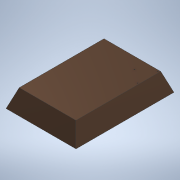
# Autodesk Inventor part: Base
Saved by Autodesk Inventor 2022 (Build 260153000, 153)
## iProperties
Created: 2021-06-28
Part Number: Base
Material: Generic
Document SubType Name: Modeling
Designer: Prajwal Patil
Density: 1 g/cm^3
Appearance: Default
Author: Prajwal Patil
Autodesk Inventor part; units mm, degrees
ref_plane "YZ Plane" through (0, 0, 0) normal (1, 0, 0) x (0, 1, 0)
ref_plane "XZ Plane" through (0, 0, 0) normal (0, 1, 0) x (-1, 0, 0)
ref_plane "XY Plane" through (0, 0, 0) normal (0, 0, 1) x (1, 0, 0)
sketch "Sketch1" plane through (0, 0, 0) normal (0, 1, 0) x (-1, 0, 0)
  line L0 (0, 0) -> (0, -129.54)
  line L1 (0, 0) -> (99.06, 0)
  line L2 (99.06, 0) -> (99.06, -129.54)
  line L3 (99.06, -129.54) -> (0, -129.54)
  line L4 (140.0707, 45.2128) -> (-215.5629, 45.2128)
  line L5 (-215.5629, 45.2128) -> (-215.5629, -504.8339)
  line L6 (-215.5629, -504.8339) -> (140.0707, -504.8339)
  line L7 (140.0707, -504.8339) -> (140.0707, 45.2128)
  dimension "d0" = 129.54
  dimension "d1" = 99.06
  constraints: 16 end point, 3 perpendicular, 2 horizontal, 2 parallel, 1 vertical
  measures "d0" distance of L0.start L0.end
  measures "d1" distance of L0.start L1.end
extrude "Extrusion1" add sketch "Sketch1" against normal blind 101.6 contours L1 L2 L3 L0 | L7 L6 L5 L4
draft "FaceDraft1" angle -20 pull direction (0, -1, 0) faces at (215.5629, -33.8667, -138.1361) (-21.5262, -33.8667, 45.2128) fixed edges at (215.5629, -101.6, -229.8106) (37.7461, -101.6, 45.2128)
draft "FaceDraft2" angle -20 pull direction (0, -1, 0) faces at (-140.0707, -67.7333, -150.4626) (84.6919, -67.7333, -504.8339) fixed edges at (-140.0707, 0, -248.3003) (37.7461, -101.6, -504.8339)
sketch "Sketch2" plane through (0, 0, 0) normal (0, 1, 0) x (1, 0, 0)
  line L0 (178.5835, 467.8546) -> (215.5629, 504.8339) projected
  line L1 (178.5835, 467.8546) -> (79.5235, 467.8546)
  line L2 (79.5235, 467.8546) -> (79.5235, 338.3146)
  line L3 (79.5235, 338.3146) -> (178.5835, 338.3146)
  line L4 (178.5835, 338.3146) -> (178.5835, 467.8546)
  line L5 (178.5835, 338.3146) -> (178.5835, 346.4426)
  line L6 (178.5835, -8.2334) -> (178.5835, 467.8546) projected
  line L7 (178.5835, 467.8546) -> (178.5835, 459.7266)
  circle A0 centre (95.5255, 403.0846) radius 2.54
  circle A1 centre (169.6935, 346.4426) radius 2.54
  circle A2 centre (169.6935, 459.7266) radius 2.54
  point P0 (0, 0)
  dimension "d6" = 99.06
  dimension "d7" = 129.54
  dimension "d13" = 5.08
  dimension "d14" = 5.08
  dimension "d15" = 5.08
  constraints: 12 end point, 3 centre point, 2 parallel, 2 point on line, 1 horizontal, 1 perpendicular
  measures "d6" distance of L3.end L2.end
  measures "d7" distance of L2.end L1.end
  measures "d13" diameter of A0
  measures "d14" diameter of A1
  measures "d15" diameter of A2
extrude "Extrusion2" cut sketch "Sketch2" against normal blind 5.08 contours A0 | A1 | A2
equation "\"d16\" = d14"
body "Solid1"
